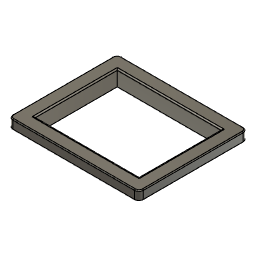
Bezel (Autodesk Fusion 360 design; units mm, degrees)
Autodesk Fusion 360 part; units mm, degrees
sketch "Sketch1" plane through (0, 0, 0) normal (0, 1, 0) x (1, 0, 0)
  line L0 (0, 0) -> (59.7, 0)
  line L1 (59.7, 0) -> (59.7, 49.7)
  line L2 (59.7, 49.7) -> (0, 49.7)
  line L3 (0, 49.7) -> (0, 0)
  line L4 (29.85, 49.7) -> (30, 0) construction
  line L5 (0, 24.85) -> (59.7, 24.85)
  line L6 (50.775, 40.7) -> (9.075, 40.7)
  line L7 (9.075, 40.7) -> (9.075, 9)
  line L8 (9.075, 9) -> (50.775, 9)
  line L9 (50.775, 9) -> (50.775, 40.7)
  line L10 (50.775, 40.7) -> (9.075, 9) construction
  line L11 (9.075, 40.7) -> (50.775, 9) construction
  circle A0 centre (3.6, 25.2) radius 0.95
  circle A1 centre (56.1, 25.2) radius 0.95
  circle A2 centre (29.85, 46.2) radius 0.95
  point P0 (29.925, 24.85)
  dimension "d1" = 59.7
  dimension "d2" = 49.7
  dimension "d5" = 41.7
  dimension "d6" = 31.7
  dimension "d7" = 1.9
  dimension "d8" = 3.6
  dimension "d9" = 25.2
  dimension "d10" = 1.9
  dimension "d11" = 3.6
  dimension "d12" = 1.9
  dimension "d13" = 3.5
  constraint horizontal L0
  constraint vertical L1
  constraint horizontal L2
  constraint vertical L3
  constraint coincident L0.start L3.end
  constraint midpoint L2 L4.start
  constraint coincident L0 L4.end
  constraint midpoint L3 L5.start
  constraint midpoint L1 L5.end
  constraint horizontal L6
  constraint perpendicular L6 L7
  constraint parallel L6 L8
  constraint parallel L7 L9
  constraint coincident L10 P0
  constraint coincident L11 P0
  constraint midpoint L4 P0
  constraint horizontal A0.centre A1.centre
  measures "d1" distance of L0.start L0.end
  measures "d2" distance of L0.start L2.end
  measures "d5" distance of L7.end L8.end
  measures "d6" distance of L6.end L7.end
  measures "d7" diameter of A0
  measures "d8" distance of L3 A0.centre
  measures "d9" distance of L0 A0.centre
  measures "d10" diameter of A1
  measures "d11" distance of L1 A1.centre
  measures "d12" diameter of A2
  measures "d13" distance of L2 A2.centre
ref_plane "WorkPlane1" through (0, 4, 0) normal (0, 1, 0) x (0, 0, 1)
sketch "Sketch2" plane through (0, 4, 0) normal (0, 1, 0) x (1, 0, 0)
  line L0 (0, 49.7) -> (0, 0)
  line L1 (59.7, 49.7) -> (0, 49.7)
  line L2 (0, 0) -> (59.7, 0)
  line L3 (59.7, 0) -> (59.7, 49.7)
  line L4 (5.875, 43.9) -> (53.975, 43.9)
  line L5 (53.975, 43.9) -> (53.975, 5.8)
  line L6 (53.975, 5.8) -> (5.875, 5.8)
  line L7 (5.875, 5.8) -> (5.875, 43.9)
  line L8 (9.075, 40.7) -> (9.075, 9)
  line L9 (50.775, 9) -> (50.775, 40.7)
  line L10 (50.775, 40.7) -> (9.075, 40.7)
  line L11 (9.075, 9) -> (50.775, 9)
  dimension "d15" = 3.2
  dimension "d16" = 3.2
  dimension "d17" = 3.2
  dimension "d18" = 3.2
  constraint horizontal L4
  constraint vertical L5
  constraint horizontal L6
  constraint vertical L7
  measures "d15" distance of L7 L8
  measures "d16" distance of L5 L9
  measures "d17" distance of L4 L10
  measures "d18" distance of L6 L11
extrude "Extrude1" add sketch "Sketch1" along normal blind 4 contours L0 L1 L3 L5 L7 L8 L9 A0 A1 | L1 L2 L3 L5 L6 L7 L9 A0 A1 | L5 A0 | L5 A0 | L5 A1 | L5 A1 | A2
loft "Loft2" cut profiles "Sketch2", "Sketch1" section 1 contours L4 L5 L6 L7 | L8 L9 L10 L11 section 2 contours L5 L6 L7 L9 | L5 L7 L8 L9
extrude "Extrude2" cut sketch "Sketch1" along normal blind 3 contours L5 A0 | L5 A0 | L5 A1 | L5 A1 | A2
fillet "Fillet1" radius 2 1 edges at (0, 2, -49.7)
fillet "Fillet1" radius 2 1 edges at (59.7, 2, -49.7)
fillet "Fillet1" radius 2 1 edges at (59.7, 2, 0)
fillet "Fillet1" radius 2 1 edges at (0, 2, 0)
fillet "Fillet2" radius 0.4 8 edges at (0.5858, 4, -49.1142) (0, 4, -24.85) (0.5858, 4, -0.5858) (29.85, 4, 0) (59.1142, 4, -0.5858) (59.7, 4, -24.85) (59.1142, 4, -49.1142) (29.85, 4, -49.7)
fillet "Fillet3" radius 1 4 edges at (29.925, 4, -43.9) (5.875, 4, -24.85) (29.925, 4, -5.8) (53.975, 4, -24.85)
loft "Loft1" [rolled back]
